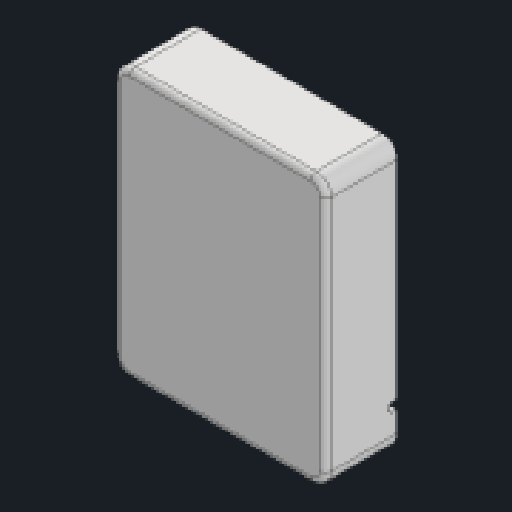
# Autodesk Inventor part: Housing
Saved by Autodesk Inventor 2026.2 (Build 302298000, 298)
## iProperties
Created: 2026-02-21
Part Number: Housing
Material: Generic
Document SubType Name: Modeling
Designer: niuke
Density: 1 g/cm^3
Appearance: Default
Author: niuke
Autodesk Inventor part; units mm, degrees
ref_plane "YZ Plane" through (0, 0, 0) normal (1, 0, 0) x (0, 1, 0)
ref_plane "XZ Plane" through (0, 0, 0) normal (0, 1, 0) x (-1, 0, 0)
ref_plane "XY Plane" through (0, 0, 0) normal (0, 0, 1) x (1, 0, 0)
ref_plane "Work Plane1" through (-101, -22.1576, 4) normal (0, 0, 1) x (1, 0, 0)
sketch "Sketch1" plane through (0, 0, 0) normal (0, 0, 1) x (1, 0, 0)
  circle A0 centre (0, 0) radius 1.375 construction
  circle A1 centre (-86, 0) radius 1.375 construction
  circle A2 centre (-86, 58) radius 1.375 construction
  circle A3 centre (0, 58) radius 1.375 construction
  line L0 (-95.4, 62) -> (3.4, 62) construction
  line L1 (-96, -16.4) -> (-96, 61.4) construction
  line L2 (4, 61.4) -> (4, -16.4) construction
  line L3 (4, 61.4) -> (4, 62) construction
  line L4 (4, 62) -> (3.4, 62) construction
  line L5 (-95.4, 62) -> (-96, 62) construction
  line L6 (-96, 62) -> (-96, 61.4) construction
  line L7 (4, -16.4) -> (4, -67.8) construction
  line L8 (4, -67.8) -> (-96, -67.8) construction
  line L9 (-96, -67.8) -> (-96, -16.4) construction
  line L10 (6, -16.4) -> (6, 61.4)
  line L11 (6, 61.4) -> (6, 64)
  line L12 (6, 64) -> (3.4, 64)
  line L13 (3.4, 64) -> (-95.4, 64)
  line L14 (-95.4, 64) -> (-98, 64)
  line L15 (-98, 64) -> (-98, 61.4)
  line L16 (-98, 61.4) -> (-98, -16.4)
  line L17 (-98, -16.4) -> (-98, -69.8)
  line L18 (-98, -69.8) -> (6, -69.8)
  line L19 (6, -69.8) -> (6, -16.4)
  line L20 (-95.4, 68) -> (3.4, 68)
  line L21 (3.4, 68) -> (10, 68)
  line L22 (10, 68) -> (10, 61.4)
  line L23 (10, 61.4) -> (10, -16.4)
  line L24 (10, -16.4) -> (10, -73.8)
  line L25 (10, -73.8) -> (-102, -73.8)
  line L26 (-102, -73.8) -> (-102, -16.4)
  line L27 (-102, -16.4) -> (-102, 61.4)
  line L28 (-102, 61.4) -> (-102, 68)
  line L29 (-102, 68) -> (-95.4, 68)
  line L30 (3.4, -17) -> (-95.4, -17) construction
  dimension "d1" = 2
  dimension "d2" = 4
  dimension "d3" = 50.8
  constraints: 54 end point, 12 perpendicular, 2 vertical, 1 horizontal, 18 other
  measures "d1" distance between parallel lines of L0 L13
  measures "d2" distance between parallel lines of L13 L20
  measures "d3" distance between parallel lines of L8 L30
extrude "Extrusion1" add sketch "Sketch1" along normal blind 4 from surface at 4 contours L19 L18 L17 L16 L15 L14 L13 L12 L11 L10 | L20 L21 L22 L23 L24 L25 L26 L27 L28 L29
sketch "Sketch3" plane through (10, 68, 4) normal (0, 0, -1) x (-1, 0, 0)
  line L0 (112, 0) -> (0, 0) projected
  line L1 (0, 0) -> (0, -141.8) projected
  line L2 (0, -141.8) -> (112, -141.8) projected
  line L3 (112, -141.8) -> (112, 0) projected
  line L4 (4, -4) -> (4, -137.8)
  line L5 (4, -137.8) -> (108, -137.8)
  line L6 (108, -137.8) -> (108, -4)
  line L7 (108, -4) -> (4, -4)
  point P0 (10, -68)
  constraints: 8 end point, 2 perpendicular, 1 parallel, 1 vertical
ref_plane "Work Plane2" through (-11.2, 28.1418, -29.8714) normal (0, 0, -1) x (-1, -0.0000063, 0)
sketch "Sketch4" plane through (10, 68, 4) normal (0, 0, -1) x (-1, 0, 0)
  circle A0 centre (10, -10) radius 1.375 construction
  circle A1 centre (10, -68) radius 1.375 construction
  circle A2 centre (96, -68) radius 1.375 construction
  circle A3 centre (96, -10) radius 1.375 construction
  circle A4 centre (96, -10) radius 1.25
  circle A5 centre (96, -68) radius 1.25
  circle A6 centre (10, -68) radius 1.25
  circle A7 centre (10, -10) radius 1.25
  circle A8 centre (10, -10) radius 3.5
  circle A9 centre (10, -68) radius 3.5
  circle A10 centre (96, -68) radius 3.5
  circle A11 centre (96, -10) radius 3.5
  dimension "d6" = 2.5
  dimension "d7" = 7
  constraints: 8 centre point, 8 coincident, 6 equal radius
  measures "d6" diameter of A7
  measures "d7" diameter of A10
ref_plane "Work Plane3" through (-96, -17, 0) normal (0, 0, 1) x (1, 0, 0)
extrude "Extrusion2" add sketch "Sketch4" along normal up to surface (4 mm away)
extrude "Extrusion3" add sketch "Sketch3" along normal up to surface (33.8714 mm away)
fillet "Fillet1" radius 2 4 edges at (3.5, 0, 4) (-82.5, 0, 4) (-82.5, 58, 4) (3.5, 58, 4)
fillet "Fillet2" radius 8 4 edges at (-102, -73.8, -10.9357) (10, -73.8, -10.9357) (-102, 68, -10.9357) (10, 68, -10.9357)
fillet "Fillet3" radius 4 4 edges at (6, 64, -12.9357) (-98, 64, -12.9357) (6, -69.8, -12.9357) (-98, -69.8, -12.9357)
sketch "Sketch5" plane through (2, -73.8, -29.8714) normal (0, 0, -1) x (-1, 0, 0)
  circle A0 centre (0, 8) radius 1.45
  circle A1 centre (0, 133.8) radius 1.45
  arc A2 (-4, 8) -> (0, 4) centre (0, 8) ccw construction
  line L0 (0, 4) -> (96, 4) projected
  line L1 (-4, 133.8) -> (-4, 8) projected
  line L2 (4, 8) -> (4, 4)
  line L3 (0, 12) -> (-4, 12)
  arc A3 (-4, 8) -> (0, 4) centre (0, 8) ccw
  arc A4 (4, 8) -> (0, 12) centre (0, 8) ccw
  arc A5 (0, 137.8) -> (-4, 133.8) centre (0, 133.8) ccw projected
  line L4 (96, 137.8) -> (0, 137.8) projected
  line L5 (-4, 129.8) -> (0, 129.8)
  arc A6 (0, 129.8) -> (4, 133.8) centre (0, 133.8) ccw
  line L6 (4, 133.8) -> (4, 137.8)
  line L7 (48, 137.8) -> (48, 4) construction
  circle A7 centre (96, 8) radius 1.45
  circle A8 centre (96, 133.8) radius 1.45
  line L8 (92, 8) -> (92, 4)
  line L9 (96, 12) -> (100, 12)
  arc A9 (96, 12) -> (92, 8) centre (96, 8) ccw
  line L10 (100, 129.8) -> (96, 129.8)
  arc A10 (92, 133.8) -> (96, 129.8) centre (96, 133.8) ccw
  line L11 (92, 133.8) -> (92, 137.8)
  line L12 (100, 8) -> (100, 133.8) projected
  arc A11 (100, 133.8) -> (96, 137.8) centre (96, 133.8) ccw projected
  arc A12 (96, 4) -> (100, 8) centre (96, 8) ccw projected
  point P0 (2, 73.8)
  point P1 (92, 137.8)
  point P2 (92, 4)
  dimension "d15" = 2.9
  constraints: 20 end point, 12 symmetric about line, 10 point on circle, 9 centre point, 4 coincident, 4 point on line, 4 tangent, 3 equal radius, 2 midpoint, 2 perpendicular, 1 horizontal, 1 vertical, 4 other
  measures "d15" diameter of A1
extrude "Extrusion4" add sketch "Sketch5" against normal blind 7 contours A3 L1 L3 A4 L2 L0 | L8 A9 L9 L12 A12 L0 | L1 A5 L4 L6 A6 L5 | L10 A10 L11 L4 A11 L12
fillet "Fillet4" radius 3 20 edges at (-96.8284, 62.8284, -22.8714) (-92, 64, -22.8714) (-98, 58, -22.8714) (4.8284, 62.8284, -22.8714) (6, 58, -22.8714) (0, 64, -22.8714) (0, -69.8, -22.8714) (6, -63.8, -22.8714) (4.8284, -68.6284, -22.8714) (-98, -63.8, -22.8714) (-92, -69.8, -22.8714) (-96.8284, -68.6284, -22.8714) (-98, -61.8, -26.3714) (-90, -69.8, -26.3714) (-2, -69.8, -26.3714) (6, -61.8, -26.3714) (6, 56, -26.3714) (-2, 64, -26.3714) (-90, 64, -26.3714) (-98, 56, -26.3714)
fillet "Fillet5" radius 3 8 edges at (7.6569, 65.6569, 8) (10, -2.9, 8) (7.6569, -71.4569, 8) (-46, -73.8, 8) (-99.6569, -71.4569, 8) (-102, -2.9, 8) (-99.6569, 65.6569, 8) (-46, 68, 8)
sketch "Sketch6" plane through (6, -65.8, 4) normal (-1, 0, 0) x (0, 0, 1)
  arc A0 (-31.3714, 10.85) -> (-31.3714, 15.85) centre (-31.3714, 13.35) ccw
  line L0 (-33.8714, 118.8) -> (-33.8714, 7) projected
  line L1 (-31.3714, 15.85) -> (-33.8714, 15.85)
  line L2 (-31.3714, 10.85) -> (-33.8714, 10.85)
  point P0 (-4, 65.8)
  dimension "d20" = 5
  dimension "d21" = 6.35
  constraints: 4 end point, 3 tangent, 2 point on circle, 2 point on line, 1 centre point, 1 horizontal, 1 perpendicular
  measures "d20" diameter of A0
  measures "d21" vertical distance of L0.end A0.centre
extrude "Extrusion5" cut sketch "Sketch6" against normal blind 7
fillet "Fillet6" radius 1 3 edges at (6, -52.45, -24.8714) (6, -54.95, -28.6214) (6, -49.95, -28.6214)
body "Solid1"
